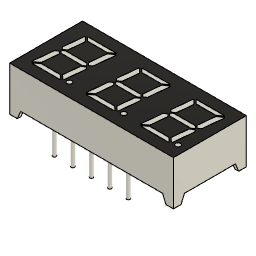
DICE_2381 (Autodesk Fusion 360 design; units mm, degrees)
Autodesk Fusion 360 part; units mm, degrees
sketch "Footprint" plane through (0, 0, 0) normal (0, 0, 1) x (1, 0, 0)
  line L0 (-11.25, 5) -> (11.25, 5)
  line L1 (11.25, 5) -> (11.25, -5)
  line L2 (11.25, -5) -> (-11.25, -5)
  line L3 (-11.25, -5) -> (-11.25, 5)
  line L4 (-11.25, 5) -> (11.25, -5) construction
  line L5 (11.25, 5) -> (-11.25, -5) construction
  dimension "d1" = 22.5
  dimension "d2" = 10
  constraint horizontal L0
  constraint perpendicular L0 L1
  constraint parallel L0 L2
  constraint parallel L1 L3
  constraint coincident L4 origin
  constraint coincident L5 origin
  measures "d1" distance of L1.end L2.end
  measures "d2" distance of L0.end L1.end
extrude "Extrude Height" add sketch "Footprint" along normal blind 5 makes body 1
sketch "Bottom Feature Profile" plane through (0, 0, 0) normal (0, 0, -1) x (1, 0, 0)
  line L0 (11.25, 5) -> (-11.25, 5)
  line L1 (-11.25, 5) -> (-11.25, -5)
  line L2 (-11.25, -5) -> (11.25, -5)
  line L3 (11.25, -5) -> (11.25, 5)
  circle A0 centre (-6.35, -3.76) radius 0.225
  circle A1 centre (-3.81, -3.76) radius 0.225
  circle A2 centre (-1.27, -3.76) radius 0.225
  circle A3 centre (1.27, -3.76) radius 0.225
  circle A4 centre (3.81, -3.76) radius 0.225
  circle A5 centre (6.35, -3.76) radius 0.225
  circle A6 centre (-6.35, 3.76) radius 0.225
  circle A7 centre (-3.81, 3.76) radius 0.225
  circle A8 centre (-1.27, 3.76) radius 0.225
  circle A9 centre (1.27, 3.76) radius 0.225
  circle A10 centre (3.81, 3.76) radius 0.225
  line L4 (-6.35, 3.76) -> (6.35, -3.76) construction
  line L5 (-11.25, 5) -> (-10.75, 5)
  line L6 (-10.75, 5) -> (-10.75, 3.5)
  line L7 (-10.75, 3.5) -> (-11.25, 3.5)
  line L8 (-11.25, 3.5) -> (-11.25, 5)
  line L9 (-11.25, 5) -> (-9.75, 5)
  line L10 (-9.75, 5) -> (-9.75, 4.5)
  line L11 (-9.75, 4.5) -> (-11.25, 4.5)
  line L12 (-11.25, 4.5) -> (-11.25, 5)
  dimension "d5" = 0.45
  dimension "d8" = 2.54
  dimension "d9" = 7.52
  dimension "d12" = 0.5
  dimension "d13" = 1.5
  dimension "d14" = 1.5
  dimension "d15" = 0.5
  constraint coincident A6.centre L4.start
  constraint coincident A5.centre L4.end
  constraint midpoint origin L4
  constraint horizontal L5
  constraint vertical L6
  constraint horizontal L7
  constraint vertical L8
  constraint coincident L0.end L1.start
  constraint horizontal L9
  constraint vertical L10
  constraint horizontal L11
  constraint vertical L12
  measures "d5" diameter of A0
  measures "d12" distance of L0.end L5.end
  measures "d13" distance of L0.end L7.end
  measures "d14" distance of L0.end L9.end
  measures "d15" distance of L0.end L11.end
extrude "Extrude Pins" add sketch "Bottom Feature Profile" along normal blind 5 contours A0 | A1 | A2 | A3 | A4 | A5 | A6 | A7 | A8 | A9 | A10 bodies 1
extrude "Extrude Foot" add sketch "Bottom Feature Profile" along normal blind 1.1 separate body contours L0 L6 L9 L10 L11 | L0 L1 L5 L6 L8 L9 L11 L12 | L1 L6 L7 L8 L11 makes body 2
sketch "Foot Cut Y" plane through (0, -5, 0) normal (0, -1, 0) x (1, 0, 0)
  line L0 (-11.25, 0) -> (11.25, 0)
  line L1 (11.25, 0) -> (11.25, 5)
  line L2 (11.25, 5) -> (-11.25, 5)
  line L3 (-11.25, 5) -> (-11.25, 0)
  line L4 (-11.25, 0) -> (-10.0594, 0) construction
  line L5 (-9.75, -1.1) -> (-11.25, -1.1)
  line L6 (-9.75, 0) -> (-10.2056, -1.1)
  line L7 (-9.75, 0) -> (-8.5594, 0) construction
  line L8 (-10.2056, -1.1) -> (-9.75, -1.1)
  line L9 (-9.75, -1.1) -> (-9.75, 0)
  point P0 (-9.75, 0)
  dimension "d24" = 112.5
  constraint horizontal L4
  constraint coincident L0.start L3.end
  constraint horizontal L7
  constraint coincident P0 L6.start
  constraint coincident L5 L6.end
  constraint coincident L5.start L8.end
  measures "d24" angle of L6 L7
extrude "Foot Cut Y (1)" cut sketch "Foot Cut Y" against normal blind 0.5 contours L5 L6 L8 L9 bodies 2
sketch "Foot Cut X" plane through (-11.25, 0, 0) normal (-1, 0, 0) x (0, -1, 0)
  line L0 (5, 0) -> (5, 5)
  line L1 (5, 5) -> (-5, 5)
  line L2 (-5, 5) -> (-5, 0)
  line L3 (-5, 0) -> (5, 0)
  line L4 (5, -1.1) -> (3.5, -1.1)
  line L5 (5, 0) -> (6.1906, 0) construction
  line L6 (3.5, 0) -> (3.9556, -1.1)
  line L7 (3.5, 0) -> (4.6906, 0) construction
  line L8 (3.9556, -1.1) -> (3.5, -1.1)
  line L9 (3.5, -1.1) -> (3.5, 0)
  point P0 (3.5, 0)
  dimension "d25" = 67.5
  constraint horizontal L5
  constraint coincident L0.start L3.end
  constraint horizontal L7
  constraint coincident P0 L6.start
  constraint coincident L4 L6.end
  constraint coincident L4.end L8.end
  measures "d25" angle of L6 L7
extrude "Foot Cut X (1)" cut sketch "Foot Cut X" against normal blind 0.5 contours L4 L6 L8 L9 bodies 2
mirror "Mirror1" about plane through (0, 0, 0) normal (1, 0, 0) of bodies 2 makes body 3
mirror "Mirror2" about plane through (0, 0, 0) normal (0, 1, 0) of bodies 2 3 makes body 4 at (-11.25, 4.1519, -0.3667) makes body 5 at (11.25, 4.1519, -0.3667)
combine "Combine1" operation add target body 1 tool bodies 2 3 4 5
sketch "Characters" plane through (0, 0, 5) normal (0, 0, 1) x (-1, 0, 0)
  line L0 (11.25, 5) -> (-11.25, 5)
  line L1 (-11.25, -5) -> (11.25, -5)
  line L2 (11.25, -5) -> (11.25, 5)
  line L3 (9.017, 2.893) -> (6.4084, 2.893)
  line L4 (6.4084, 2.893) -> (5.806, 3.4413)
  line L5 (5.806, 3.4413) -> (5.8789, 3.5021)
  line L6 (5.8789, 3.5021) -> (9.667, 3.5021)
  line L7 (9.667, 3.5021) -> (9.7372, 3.4435)
  line L8 (9.7372, 3.4435) -> (9.017, 2.893)
  line L9 (5.1412, -3.502) -> (5.0941, -3.4552)
  line L10 (5.0941, -3.4552) -> (5.8183, -2.9484)
  line L11 (5.8183, -2.9484) -> (8.5135, -2.9484)
  line L12 (8.5135, -2.9484) -> (9.0235, -3.4552)
  line L13 (9.0235, -3.4552) -> (8.9565, -3.502)
  line L14 (8.9565, -3.502) -> (5.1412, -3.502)
  line L15 (9.8988, 3.3087) -> (9.9574, 3.2598)
  line L16 (9.9574, 3.2598) -> (9.6615, 0.4384)
  line L17 (9.6615, 0.4384) -> (9.2659, 0.1616)
  line L18 (9.2659, 0.1616) -> (8.934, 0.4915)
  line L19 (8.934, 0.4915) -> (9.1712, 2.7527)
  line L20 (9.1712, 2.7527) -> (9.8988, 3.3087)
  line L21 (5.1781, -0.3717) -> (5.5451, -0.1149)
  line L22 (5.5451, -0.1149) -> (5.901, -0.4686)
  line L23 (5.901, -0.4686) -> (5.6549, -2.8143)
  line L24 (5.6549, -2.8143) -> (4.9474, -3.3094)
  line L25 (4.9474, -3.3094) -> (4.8772, -3.2396)
  line L26 (4.8772, -3.2396) -> (5.1781, -0.3717)
  line L27 (6.0052, 0.525) -> (5.5256, 0.1894)
  line L28 (5.5256, 0.1894) -> (5.2642, 0.4492)
  line L29 (5.2642, 0.4492) -> (5.5562, 3.2329)
  line L30 (5.5562, 3.2329) -> (5.6445, 3.3065)
  line L31 (5.6445, 3.3065) -> (6.2401, 2.7644)
  line L32 (6.2401, 2.7644) -> (6.0052, 0.525)
  line L33 (9.2434, -0.0529) -> (8.8838, -0.3045)
  line L34 (8.8838, -0.3045) -> (5.9742, -0.3045)
  line L35 (5.9742, -0.3045) -> (5.6147, 0.0529)
  line L36 (5.6147, 0.0529) -> (5.9742, 0.3046)
  line L37 (5.9742, 0.3046) -> (8.8838, 0.3046)
  line L38 (8.8838, 0.3046) -> (9.2434, -0.0529)
  line L39 (8.8253, -0.5442) -> (9.2696, -0.2333)
  line L40 (9.2696, -0.2333) -> (9.5607, -0.5225)
  line L41 (9.5607, -0.5225) -> (9.2712, -3.2819)
  line L42 (9.2712, -3.2819) -> (9.1983, -3.3329)
  line L43 (9.1983, -3.3329) -> (8.5956, -2.7339)
  line L44 (8.5956, -2.7339) -> (8.8253, -0.5442)
  line L45 (-5.9022, 2.893) -> (-8.5108, 2.893)
  line L46 (-8.5108, 2.893) -> (-9.1132, 3.4413)
  line L47 (-9.1132, 3.4413) -> (-9.0402, 3.5021)
  line L48 (-9.0402, 3.5021) -> (-5.2522, 3.5021)
  line L49 (-5.2522, 3.5021) -> (-5.1819, 3.4435)
  line L50 (-5.1819, 3.4435) -> (-5.9022, 2.893)
  line L51 (-9.7779, -3.502) -> (-9.825, -3.4552)
  line L52 (-9.825, -3.4552) -> (-9.1008, -2.9484)
  line L53 (-9.1008, -2.9484) -> (-6.4056, -2.9484)
  line L54 (-6.4056, -2.9484) -> (-5.8957, -3.4552)
  line L55 (-5.8957, -3.4552) -> (-5.9626, -3.502)
  line L56 (-5.9626, -3.502) -> (-9.7779, -3.502)
  line L57 (-5.0204, 3.3087) -> (-4.9617, 3.2598)
  line L58 (-4.9617, 3.2598) -> (-5.2577, 0.4384)
  line L59 (-5.2577, 0.4384) -> (-5.6533, 0.1616)
  line L60 (-5.6533, 0.1616) -> (-5.9852, 0.4915)
  line L61 (-5.9852, 0.4915) -> (-5.748, 2.7527)
  line L62 (-5.748, 2.7527) -> (-5.0204, 3.3087)
  line L63 (-9.7411, -0.3717) -> (-9.3741, -0.1149)
  line L64 (-9.3741, -0.1149) -> (-9.0182, -0.4686)
  line L65 (-9.0182, -0.4686) -> (-9.2643, -2.8143)
  line L66 (-9.2643, -2.8143) -> (-9.9717, -3.3094)
  line L67 (-9.9717, -3.3094) -> (-10.042, -3.2396)
  line L68 (-10.042, -3.2396) -> (-9.7411, -0.3717)
  line L69 (-8.914, 0.525) -> (-9.3935, 0.1894)
  line L70 (-9.3935, 0.1894) -> (-9.655, 0.4492)
  line L71 (-9.655, 0.4492) -> (-9.363, 3.2329)
  line L72 (-9.363, 3.2329) -> (-9.2747, 3.3065)
  line L73 (-9.2747, 3.3065) -> (-8.6791, 2.7644)
  line L74 (-8.6791, 2.7644) -> (-8.914, 0.525)
  line L75 (-5.6758, -0.0529) -> (-6.0354, -0.3045)
  line L76 (-6.0354, -0.3045) -> (-8.9449, -0.3045)
  line L77 (-8.9449, -0.3045) -> (-9.3045, 0.0529)
  line L78 (-9.3045, 0.0529) -> (-8.9449, 0.3046)
  line L79 (-8.9449, 0.3046) -> (-6.0354, 0.3046)
  line L80 (-6.0354, 0.3046) -> (-5.6758, -0.0529)
  line L81 (-6.0939, -0.5442) -> (-5.6495, -0.2333)
  line L82 (-5.6495, -0.2333) -> (-5.3585, -0.5225)
  line L83 (-5.3585, -0.5225) -> (-5.648, -3.2819)
  line L84 (-5.648, -3.2819) -> (-5.7209, -3.3329)
  line L85 (-5.7209, -3.3329) -> (-6.3236, -2.7339)
  line L86 (-6.3236, -2.7339) -> (-6.0939, -0.5442)
  line L87 (1.5574, 2.893) -> (-1.0512, 2.893)
  line L88 (-1.0512, 2.893) -> (-1.6536, 3.4413)
  line L89 (-1.6536, 3.4413) -> (-1.5807, 3.5021)
  line L90 (-1.5807, 3.5021) -> (2.2074, 3.5021)
  line L91 (2.2074, 3.5021) -> (2.2777, 3.4435)
  line L92 (2.2777, 3.4435) -> (1.5574, 2.893)
  line L93 (-2.3183, -3.502) -> (-2.3655, -3.4552)
  line L94 (-2.3655, -3.4552) -> (-1.6412, -2.9484)
  line L95 (-1.6412, -2.9484) -> (1.054, -2.9484)
  line L96 (1.054, -2.9484) -> (1.5639, -3.4552)
  line L97 (1.5639, -3.4552) -> (1.4969, -3.502)
  line L98 (1.4969, -3.502) -> (-2.3183, -3.502)
  line L99 (2.4392, 3.3087) -> (2.4979, 3.2598)
  line L100 (2.4979, 3.2598) -> (2.2019, 0.4384)
  line L101 (2.2019, 0.4384) -> (1.8063, 0.1616)
  line L102 (1.8063, 0.1616) -> (1.4744, 0.4915)
  line L103 (1.4744, 0.4915) -> (1.7116, 2.7527)
  line L104 (1.7116, 2.7527) -> (2.4392, 3.3087)
  line L105 (-2.2815, -0.3717) -> (-1.9145, -0.1149)
  line L106 (-1.9145, -0.1149) -> (-1.5586, -0.4686)
  line L107 (-1.5586, -0.4686) -> (-1.8047, -2.8143)
  line L108 (-1.8047, -2.8143) -> (-2.5122, -3.3094)
  line L109 (-2.5122, -3.3094) -> (-2.5824, -3.2396)
  line L110 (-2.5824, -3.2396) -> (-2.2815, -0.3717)
  line L111 (-1.4544, 0.525) -> (-1.9339, 0.1894)
  line L112 (-1.9339, 0.1894) -> (-2.1954, 0.4492)
  line L113 (-2.1954, 0.4492) -> (-1.9034, 3.2329)
  line L114 (-1.9034, 3.2329) -> (-1.8151, 3.3065)
  line L115 (-1.8151, 3.3065) -> (-1.2195, 2.7644)
  line L116 (-1.2195, 2.7644) -> (-1.4544, 0.525)
  line L117 (1.7838, -0.0529) -> (1.4242, -0.3045)
  line L118 (1.4242, -0.3045) -> (-1.4853, -0.3045)
  line L119 (-1.4853, -0.3045) -> (-1.8449, 0.0529)
  line L120 (-1.8449, 0.0529) -> (-1.4853, 0.3046)
  line L121 (-1.4853, 0.3046) -> (1.4242, 0.3046)
  line L122 (1.4242, 0.3046) -> (1.7838, -0.0529)
  line L123 (1.3657, -0.5442) -> (1.8101, -0.2333)
  line L124 (1.8101, -0.2333) -> (2.1011, -0.5225)
  line L125 (2.1011, -0.5225) -> (1.8116, -3.2819)
  line L126 (1.8116, -3.2819) -> (1.7387, -3.3329)
  line L127 (1.7387, -3.3329) -> (1.136, -2.7339)
  line L128 (1.136, -2.7339) -> (1.3657, -0.5442)
  line L129 (12.3915, -4.5932) -> (-12.3915, 4.5932) construction
  line L130 (-12.3915, -4.5932) -> (12.3915, 4.5932) construction
  circle A0 centre (4.8772, 3.1599) radius 0.3418
  circle A1 centre (-2.5824, 3.1598) radius 0.3421
  circle A2 centre (-10.042, 3.1595) radius 0.3426
  constraint midpoint L130 origin
extrude "Indent LED" cut sketch "Characters" against normal blind 0.01 bodies 1
ref_plane "WorkPlane1" through (-10.7278, -4.4778, -4.2) normal (0, 0, -1) x (-1, 0, 0)
extrude "Trim Leads" cut 11 faces at (-6.3844, -3.6989, -5) (-3.892, -3.8533, -5) (-1.2451, -3.6793, -5) (1.2949, -3.6793, -5) (3.7441, -3.7636, -5) (6.3156, 3.8211, -5) (3.7441, 3.7564, -5) (1.2949, 3.8407, -5) (-1.2451, 3.8407, -5) (-3.892, 3.6667, -5) (-6.3844, 3.8211, -5) along direction (0, 0, -1) up to surface end surface through (-10.7278, -4.4778, -4.2) normal (0, 0, -1) offset 0 on bodies 1 bodies 1
sketch "Pin Origin Reference" plane through (0, 0, -1.1) normal (0, 0, -1) x (1, 0, 0)
  circle A0 centre (-6.35, 3.76) radius 0.225
  point P0 (-6.35, 3.76)
  constraint coincident P0 A0.centre
move_body "Move1" bodies 1 to x (1, 0, 0) y (0, 1, 0) z (0, 0, 1) at (6.35, 3.76, 1.1)
equation "d24 = 90 deg + 22.5 deg"
equation "d25 = 90 deg - 22.5 deg"
equation "segment_d = 0.01 mm" comment "Distance segments are cut into surface"
equation "d32 = -segment_d"
equation "pcb_t = 1.6 mm" comment "PCB thickness (used to trim pins)"
equation "d35 = pcb_t + lead_surplus"
equation "lead_surplus = 1.5 mm" comment "Length the pins extend past the bottom of the PCB"
named bodies: "Dice", "Foot", "Foot (1)", "Foot (2)", "Foot (1) (1)"
